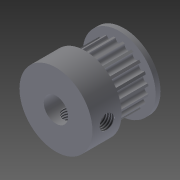
# Autodesk Inventor part: PulleyGT2x20tx5mmBore
Saved by Autodesk Inventor 2015 (Build 190159000, 159)
## iProperties
Company: RobotDigg
Created: 2014-01-11
Part Number: PulleyGT2x20tx5mmBore
Material: Generic
Document SubType Name: Modeling
Designer: Jack
Density: 1 g/cm^3
Appearance: Default
Author: Jack
Autodesk Inventor part; units mm, degrees
ref_plane "YZ Plane" through (0, 0, 0) normal (1, 0, 0) x (0, 1, 0)
ref_plane "XZ Plane" through (0, 0, 0) normal (0, 1, 0) x (-1, 0, 0)
ref_plane "XY Plane" through (0, 0, 0) normal (0, 0, 1) x (1, 0, 0)
sketch "Sketch1" plane through (0, 0, 0) normal (0, 1, 0) x (-1, 0, 0)
  circle A0 centre (0, 0) radius 7.5
  dimension "d0" = 15
  constraints: 1 centre point, 1 coincident
  measures "d0" diameter of A0
extrude "Extrusion1" add sketch "Sketch1" along normal blind 6
sketch "Sketch2" plane through (0, 6, 0) normal (0, 1, 0) x (1, 0, 0)
  circle A0 centre (0, 0) radius 7.5 projected
  line L0 (0, -7.5) -> (0, 7.5) construction
  line L1 (0.7, 6) -> (0.7, 5.9)
  line L2 (-0.7, 6) -> (-0.7, 5.9)
  arc A1 (-0.7, 5.9) -> (0.7, 5.9) centre (0, 5.9) ccw
  line L3 (-1.1884, 5.9227) -> (-1.1575, 5.8275)
  line L4 (-2.5198, 5.49) -> (-2.4889, 5.3949)
  arc A2 (-2.4889, 5.3949) -> (-1.1575, 5.8275) centre (-1.8232, 5.6112) ccw
  line L5 (-2.9604, 5.2656) -> (-2.9016, 5.1846)
  line L6 (-4.093, 4.4427) -> (-4.0342, 4.3618)
  arc A3 (-4.0342, 4.3618) -> (-2.9016, 5.1846) centre (-3.4679, 4.7732) ccw
  line L7 (-4.4427, 4.093) -> (-4.3618, 4.0342)
  line L8 (-5.2656, 2.9604) -> (-5.1846, 2.9016)
  arc A4 (-5.1846, 2.9016) -> (-4.3618, 4.0342) centre (-4.7732, 3.4679) ccw
  line L9 (-5.49, 2.5198) -> (-5.3949, 2.4889)
  line L10 (-5.9227, 1.1884) -> (-5.8275, 1.1575)
  arc A5 (-5.8275, 1.1575) -> (-5.3949, 2.4889) centre (-5.6112, 1.8232) ccw
  line L11 (-6, 0.7) -> (-5.9, 0.7)
  line L12 (-6, -0.7) -> (-5.9, -0.7)
  arc A6 (-5.9, -0.7) -> (-5.9, 0.7) centre (-5.9, 0) ccw
  line L13 (-5.9227, -1.1884) -> (-5.8275, -1.1575)
  line L14 (-5.49, -2.5198) -> (-5.3949, -2.4889)
  arc A7 (-5.3949, -2.4889) -> (-5.8275, -1.1575) centre (-5.6112, -1.8232) ccw
  line L15 (-5.2656, -2.9604) -> (-5.1846, -2.9016)
  line L16 (-4.4427, -4.093) -> (-4.3618, -4.0342)
  arc A8 (-4.3618, -4.0342) -> (-5.1846, -2.9016) centre (-4.7732, -3.4679) ccw
  line L17 (-4.093, -4.4427) -> (-4.0342, -4.3618)
  line L18 (-2.9604, -5.2656) -> (-2.9016, -5.1846)
  arc A9 (-2.9016, -5.1846) -> (-4.0342, -4.3618) centre (-3.4679, -4.7732) ccw
  line L19 (-2.5198, -5.49) -> (-2.4889, -5.3949)
  line L20 (-1.1884, -5.9227) -> (-1.1575, -5.8275)
  arc A10 (-1.1575, -5.8275) -> (-2.4889, -5.3949) centre (-1.8232, -5.6112) ccw
  line L21 (-0.7, -6) -> (-0.7, -5.9)
  line L22 (0.7, -6) -> (0.7, -5.9)
  arc A11 (0.7, -5.9) -> (-0.7, -5.9) centre (0, -5.9) ccw
  line L23 (1.1884, -5.9227) -> (1.1575, -5.8275)
  line L24 (2.5198, -5.49) -> (2.4889, -5.3949)
  arc A12 (2.4889, -5.3949) -> (1.1575, -5.8275) centre (1.8232, -5.6112) ccw
  line L25 (2.9604, -5.2656) -> (2.9016, -5.1846)
  line L26 (4.093, -4.4427) -> (4.0342, -4.3618)
  arc A13 (4.0342, -4.3618) -> (2.9016, -5.1846) centre (3.4679, -4.7732) ccw
  line L27 (4.4427, -4.093) -> (4.3618, -4.0342)
  line L28 (5.2656, -2.9604) -> (5.1846, -2.9016)
  arc A14 (5.1846, -2.9016) -> (4.3618, -4.0342) centre (4.7732, -3.4679) ccw
  line L29 (5.49, -2.5198) -> (5.3949, -2.4889)
  line L30 (5.9227, -1.1884) -> (5.8275, -1.1575)
  arc A15 (5.8275, -1.1575) -> (5.3949, -2.4889) centre (5.6112, -1.8232) ccw
  line L31 (6, -0.7) -> (5.9, -0.7)
  line L32 (6, 0.7) -> (5.9, 0.7)
  arc A16 (5.9, 0.7) -> (5.9, -0.7) centre (5.9, 0) ccw
  line L33 (5.9227, 1.1884) -> (5.8275, 1.1575)
  line L34 (5.49, 2.5198) -> (5.3949, 2.4889)
  arc A17 (5.3949, 2.4889) -> (5.8275, 1.1575) centre (5.6112, 1.8232) ccw
  line L35 (5.2656, 2.9604) -> (5.1846, 2.9016)
  line L36 (4.4427, 4.093) -> (4.3618, 4.0342)
  arc A18 (4.3618, 4.0342) -> (5.1846, 2.9016) centre (4.7732, 3.4679) ccw
  line L37 (4.093, 4.4427) -> (4.0342, 4.3618)
  line L38 (2.9604, 5.2656) -> (2.9016, 5.1846)
  arc A19 (2.9016, 5.1846) -> (4.0342, 4.3618) centre (3.4679, 4.7732) ccw
  line L39 (2.5198, 5.49) -> (2.4889, 5.3949)
  line L40 (1.1884, 5.9227) -> (1.1575, 5.8275)
  arc A20 (1.1575, 5.8275) -> (2.4889, 5.3949) centre (1.8232, 5.6112) ccw
  line L41 (-2.9604, 5.2656) -> (-2.5198, 5.49)
  line L42 (-1.1884, 5.9227) -> (-0.7, 6)
  line L43 (0.7, 6) -> (1.1884, 5.9227)
  line L44 (2.5198, 5.49) -> (2.9604, 5.2656)
  line L45 (4.093, 4.4427) -> (4.4427, 4.093)
  line L46 (5.2656, 2.9604) -> (5.49, 2.5198)
  line L47 (5.9227, 1.1884) -> (6, 0.7)
  line L48 (6, -0.7) -> (5.9227, -1.1884)
  line L49 (5.2656, -2.9604) -> (5.49, -2.5198)
  line L50 (4.4427, -4.093) -> (4.093, -4.4427)
  line L51 (2.9604, -5.2656) -> (2.5198, -5.49)
  line L52 (1.1884, -5.9227) -> (0.7, -6)
  line L53 (-0.7, -6) -> (-1.1884, -5.9227)
  line L54 (-2.5198, -5.49) -> (-2.9604, -5.2656)
  line L55 (-4.093, -4.4427) -> (-4.4427, -4.093)
  line L56 (-5.49, -2.5198) -> (-5.2656, -2.9604)
  line L57 (-5.9227, -1.1884) -> (-6, -0.7)
  line L58 (-6, 0.7) -> (-5.9227, 1.1884)
  line L59 (-5.49, 2.5198) -> (-5.2656, 2.9604)
  line L60 (-4.4427, 4.093) -> (-4.093, 4.4427)
  point P0 (-5.9, 0)
  dimension "d10" = 0.7
  dimension "d11" = 0.7
  dimension "d12" = 6
  dimension "d15" = 0.1
  dimension "d16" = 0.7
  dimension "d17" = 0.1
  dimension "d24" = 360
  constraints: 122 end point, 42 point on circle, 20 centre point, 20 coincident, 15 perpendicular, 2 parallel, 1 midpoint, 1 point on line, 1 vertical, 181 other
  measures "d10" distance between parallel lines of L0 L2
  measures "d11" distance between parallel lines of L0 L1
  measures "d12" vertical distance of A0.centre L2.start
  measures "d15" vertical distance of L1.start point (0, 5.9)
  measures "d16" radius of A1
  measures "d17" distance of L2.start L2.end
extrude "Extrusion2" add sketch "Sketch2" along normal blind 7 contours L43 L40 A20 L39 L44 L38 A19 L37 L45 L36 A18 L35 L46 L34 A17 L33 L47 L32 A16 L31 L48 L30 A15 L29 L49 L28 A14 L27 L50 L26 A13 L25 L51 L24 A12 L23 L52 L22 A11 L21 L53 L20 A10 L19 L54 L18 A9 L17 L55 L16 A8 L15 L56 L14 A7 L13 L57 L12 A6 L11 L58 L10 A5 L9 L59 L8 A4 L7 L60 L6 A3 L5 L41 L4 A2 L3 L42 L2 A1 L1
sketch "Sketch3" plane through (0, 13, 0) normal (0, 1, 0) x (1, 0, 0)
  circle A0 centre (0, 0) radius 7.5
  dimension "d28" = 15
  constraints: 1 centre point, 1 coincident
  measures "d28" diameter of A0
extrude "Extrusion3" add sketch "Sketch3" along normal blind 1
sketch "Sketch4" plane through (0, 0, 0) normal (0, -1, 0) x (1, 0, 0)
  circle A0 centre (0, 0) radius 7.5 projected
  circle A1 centre (0, 0) radius 2.5
  dimension "d31" = 5
  constraints: 1 centre point, 1 coincident
  measures "d31" diameter of A1
extrude "Extrusion4" cut sketch "Sketch4" against normal blind 14 contours A1
ref_plane "Work Plane4" through (7.5, 14, 0) normal (1, 0, 0) x (0, 1, 0)
ref_plane "Work Plane5" through (0, 14, -7.5) normal (0, 0, -1) x (-1, 0, 0)
sketch "Sketch9" plane through (7.5, 14, 0) normal (1, 0, 0) x (0, 1, 0)
  circle A0 centre (-11, 0) radius 1.5
  line L0 (-14, 7.5) -> (-14, -7.5) projected
  point P0 (-14, 0)
  point P1 (-14, 0)
  dimension "d47" = 3
  dimension "d48" = 3
  constraints: 1 centre point, 1 horizontal alignment, 1 midpoint
  measures "d47" diameter of A0
  measures "d48" distance from line of L0 A0.centre
extrude "Extrusion7" cut sketch "Sketch9" against normal blind 5.75
sketch "Sketch10" plane through (0, 14, -7.5) normal (0, 0, -1) x (-1, 0, 0)
  circle A0 centre (0, -11) radius 1.5
  point P0 (0, -14)
  dimension "d51" = 3
  dimension "d52" = 3
  constraints: 1 centre point, 1 vertical alignment
  measures "d51" diameter of A0
  measures "d52" distance of point (0, -14) A0.centre
extrude "Extrusion8" cut sketch "Sketch10" against normal blind 6
thread "Thread3" size "M3x0.5" class "6H" standard "ANSI Metric M Profile" full length
thread "Thread4" size "M3x0.5" class "6H" standard "ANSI Metric M Profile" full length
body "Solid1"
